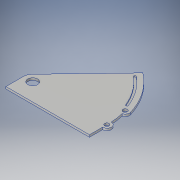
# Autodesk Inventor part: Hood panel
Saved by Autodesk Inventor 2018 (Build 220112000, 112)
## iProperties
Created: 2020-01-18
Part Number: Hood panel
Material: Aluminum 6061
Document SubType Name: Modeling
Designer: Victor
Density: 2.7 g/cm^3
Appearance: Aluminum - Flat
Author: Victor
Autodesk Inventor part; units mm, degrees
ref_plane "YZ Plane" through (0, 0, 0) normal (1, 0, 0) x (0, 1, 0)
ref_plane "XZ Plane" through (0, 0, 0) normal (0, 1, 0) x (-1, 0, 0)
ref_plane "XY Plane" through (0, 0, 0) normal (0, 0, 1) x (1, 0, 0)
sketch "Sketch1" plane through (0, 0, 0) normal (0, 1, 0) x (-1, 0, 0)
  circle A0 centre (254, -50.8) radius 14.2875
  arc A1 (38.4735, -38.1055) -> (38.4735, -63.4945) centre (38.1, -50.8) ccw
  line L0 (280.9875, -50.8) -> (280.9875, 0)
  line L1 (280.9875, 0) -> (280.9875, -50.8)
  line L2 (280.9875, 0) -> (38.1, 0)
  line L3 (38.1, -38.1) -> (38.1, 0)
  arc A2 (38.4735, -63.4945) -> (43.8871, -100.4525) centre (254, -50.8) ccw
  arc A3 (51.1687, -124.7749) -> (66.9545, -158.6276) centre (254, -50.8) ccw
  arc A4 (80.906, -179.8398) -> (105.7377, -207.743) centre (254, -50.8) ccw
  arc A5 (273.4803, -69.4773) -> (280.9875, -50.8) centre (254, -50.8) ccw
  line L4 (125.2338, -224.0976) -> (273.4803, -69.4773)
  line L5 (280.9875, 0) -> (38.1, 0)
  line L6 (38.1, 0) -> (38.1, -38.1)
  line L7 (280.9875, 0) -> (280.9875, -50.8)
  circle A6 centre (47.1701, -112.7208) radius 6.35
  circle A7 centre (38.1, -50.8) radius 6.35
  arc A8 (43.8871, -100.4525) -> (51.1687, -124.7749) centre (47.1701, -112.7208) ccw
  arc A9 (38.4735, -38.1055) -> (38.4735, -63.4945) centre (38.1, -50.8) ccw
  arc A10 (43.8871, -100.4525) -> (51.1687, -124.7749) centre (47.1701, -112.7208) ccw
  line L8 (38.1, 0) -> (50.8, 0)
  line L9 (38.4739, -38.1) -> (38.1, -38.1)
  line L10 (38.1, -38.1) -> (38.1, 0)
  circle A11 centre (254, -50.8) radius 14.2875
  circle A12 centre (47.1701, -112.7208) radius 6.35
  circle A13 centre (38.1, -50.8) radius 6.35
  arc A14 (51.1687, -124.7749) -> (125.2338, -224.0976) centre (254, -50.8) ccw
  arc A15 (38.1934, -57.1493) -> (43.8871, -100.4525) centre (254, -50.8) ccw
  arc A16 (35.0036, -116.3632) -> (116.3789, -233.3332) centre (254, -50.8) ccw
  line L11 (125.2338, -224.0976) -> (116.3789, -233.3332)
  point P0 (0, 0)
  point P1 (44.1616, 0)
  point P2 (38.1934, -44.4507)
  dimension "d4" = 28.575
  dimension "d32" = 25.4
  dimension "d36" = 50.8
  dimension "d74" = 53.975
  dimension "d79" = 12.7
  dimension "d83" = 26.9875
  constraints: 28 point on circle, 24 end point, 17 centre point, 10 coincident, 3 collinear, 2 horizontal, 2 tangent, 1 parallel, 1 perpendicular, 1 point on line, 1 vertical
  measures "d4" diameter of A0
  measures "d32" diameter of A1
  measures "d36" distance of L0.start L0.end
  measures "d74" diameter of A5
  measures "d79" diameter of A7
  measures "d83" distance from line of L0 A0.centre
ref_plane "Work Plane1" through (0, 6.35, 0) normal (0, 1, 0) x (1, 0, 0)
extrude "Extrusion7" add sketch "Sketch1" along normal blind 6.35
sketch "Sketch4" plane through (0, 6.35, 0) normal (0, 1, 0) x (1, 0, 0)
  arc A0 (-116.4883, 215.1788) -> (-120.5628, 210.3083) centre (-118.5256, 212.7436) ccw projected
  arc A1 (-116.4883, 215.1788) -> (-120.5628, 210.3083) centre (-118.5256, 212.7436) ccw
  arc A2 (-60.849, 127.8786) -> (-54.9513, 130.2322) centre (-57.9002, 129.0554) ccw projected
  arc A3 (-60.849, 127.8786) -> (-54.9513, 130.2322) centre (-57.9002, 129.0554) ccw
  circle A4 centre (-254, 50.8) radius 14.2875 projected
  arc A5 (-54.9513, 130.2322) -> (-116.4883, 215.1788) centre (-254, 50.8) ccw projected
  arc A6 (-54.9513, 130.2322) -> (-116.4883, 215.1788) centre (-254, 50.8) ccw
  arc A7 (-60.849, 127.8786) -> (-120.5628, 210.3083) centre (-254, 50.8) ccw
  point P0 (0, 0)
  constraints: 8 point on circle, 4 centre point, 4 coincident
extrude "Extrusion9" cut sketch "Sketch4" against normal blind 3.175 contours A5 A2 A7 A0
body "Solid4"
